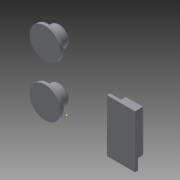
# Autodesk Inventor part: ESP_DISP_BUT
Saved by Autodesk Inventor 2015 (Build 190159000, 159)
## iProperties
Created: 2018-04-05
Part Number: ESP_DISP_BUT
Material: Типовые
Document SubType Name: Modeling
Designer: JOK
Density: 1 g/cm^3
Appearance: По умолчанию
Author: JOK
Autodesk Inventor part; units mm, degrees
ref_plane "YZ Plane" through (0, 0, 0) normal (1, 0, 0) x (0, 1, 0)
ref_plane "XZ Plane" through (0, 0, 0) normal (0, 1, 0) x (-1, 0, 0)
ref_plane "XY Plane" through (0, 0, 0) normal (0, 0, 1) x (1, 0, 0)
sketch "Эскиз1" plane through (0, 0, 0) normal (0, 1, 0) x (-1, 0, 0)
  circle A0 centre (2, 5) radius 5
  circle A1 centre (2, 21.4199) radius 5
  line L0 (-18, 0) -> (-27, 0)
  line L1 (-27, 0) -> (-27, 17)
  line L2 (-27, 17) -> (-18, 17)
  line L3 (-18, 17) -> (-18, 0)
  point P0 (0, 0)
  dimension "d0" = 10
  dimension "d1" = 10
  dimension "d2" = 9
  dimension "d3" = 17
  constraints: 8 end point, 2 centre point, 2 parallel, 1 horizontal, 1 perpendicular
  measures "d0" diameter of A0
  measures "d1" diameter of A1
  measures "d2" distance of L1.end L2.end
  measures "d3" distance of L0.end L1.end
extrude "Выдавливание1" add sketch "Эскиз1" along normal blind 1
sketch "Эскиз2" plane through (-2, 1, 21.4199) normal (0, 1, 0) x (1, 0, 0)
  circle A0 centre (0, 0) radius 5 projected
  circle A1 centre (0, 0) radius 3.25
  circle A2 centre (0, 16.4199) radius 5 projected
  line L0 (0, 11.4199) -> (0, 21.4199)
  circle A3 centre (0, 16.4199) radius 3.25
  line L1 (20, 4.4199) -> (29, 4.4199) projected
  line L2 (24.5, 4.4199) -> (24.5, 21.4199)
  line L3 (29, 21.4199) -> (20, 21.4199) projected
  line L4 (21.75, 6.1699) -> (27.25, 6.1699)
  line L5 (27.25, 6.1699) -> (27.25, 19.6699)
  line L6 (27.25, 19.6699) -> (21.75, 19.6699)
  line L7 (21.75, 19.6699) -> (21.75, 6.1699)
  line L8 (21.75, 6.1699) -> (27.25, 19.6699) construction
  line L9 (27.25, 6.1699) -> (21.75, 19.6699) construction
  point P0 (2, 21.4199)
  point P1 (24.5, 12.9199)
  dimension "d6" = 6.5
  dimension "d7" = 6.5
  dimension "d8" = 5.5
  dimension "d9" = 13.5
  constraints: 16 end point, 5 midpoint, 2 centre point, 2 coincident, 2 parallel, 2 point on circle, 1 horizontal, 1 perpendicular, 1 vertical
  measures "d6" diameter of A1
  measures "d7" diameter of A3
  measures "d8" distance of L6.end L5.end
  measures "d9" distance of L5.end L4.end
extrude "Выдавливание2" add sketch "Эскиз2" along normal blind 4 contours A1 | A3 L0 | L0 A3 | L4 L7 L6 L2 | L2 L6 L5 L4
fillet "Сопряжение1" radius 1 6 edges at (-5.25, 5, 5) (-5.25, 5, 21.4199) (25.25, 5, 8.5) (22.5, 5, 15.25) (19.75, 5, 8.5) (22.5, 5, 1.75)
sketch "Эскиз3" plane through (-2, 5, 21.4199) normal (0, 1, 0) x (1, 0, 0)
  line L0 (22.75, 7.1699) -> (22.75, 18.6699) projected
  line L1 (26.25, 7.1699) -> (22.75, 7.1699) projected
  line L2 (26.25, 18.6699) -> (26.25, 7.1699) projected
  line L3 (22.75, 18.6699) -> (26.25, 18.6699) projected
  line L4 (23.0928, 7.1539) -> (23.0928, 18.4151) construction
  line L5 (23.0928, 18.4151) -> (25.6461, 18.4151) construction
  line L6 (25.6461, 18.4151) -> (25.6461, 7.1539) construction
  line L7 (25.6461, 7.1539) -> (23.0928, 7.1539) construction
  point P0 (2, 21.4199)
  constraints: 2 other
